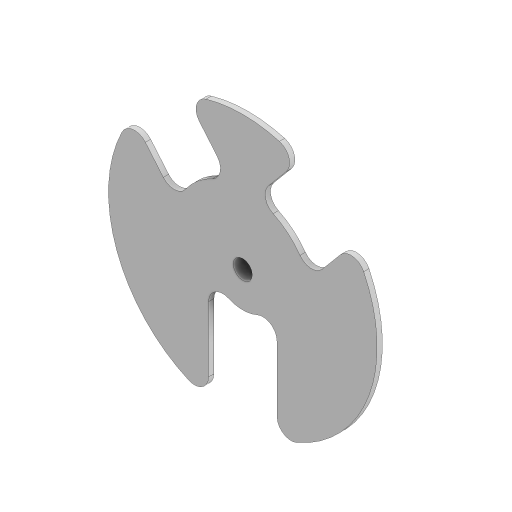
# Autodesk Inventor part: LED Diffuser
Saved by Autodesk Inventor 2024 (Build 280153000, 153)
## iProperties
Created: 2025-04-26
Part Number: LED Diffuser
Material: Generic
Document SubType Name: Modeling
Designer: Binara
Density: 1 g/cm^3
Appearance: Default
Author: Binara
Autodesk Inventor part; units mm, degrees
ref_plane "YZ Plane" through (0, 0, 0) normal (1, 0, 0) x (0, 1, 0)
ref_plane "XZ Plane" through (0, 0, 0) normal (0, 1, 0) x (-1, 0, 0)
ref_plane "XY Plane" through (0, 0, 0) normal (0, 0, 1) x (1, 0, 0)
sketch "Sketch1" plane through (0, 0, 0) normal (0, 0, 1) x (1, 0, 0)
  arc A0 (7.3638, -36.4581) -> (12.7537, -40.2088) centre (11.3638, -36.4581) ccw
  arc A1 (12.7537, -40.2088) -> (35.5951, 21.83) centre (-2.3616, 0.5806) ccw
  arc A2 (35.5951, 21.83) -> (29.0406, 22.4471) centre (32.1048, 19.876) ccw
  line L0 (29.0406, 22.4471) -> (20.2358, 11.954)
  arc A3 (13.9161, 12.201) -> (20.2358, 11.954) centre (17.1717, 14.5251) ccw
  arc A4 (13.9161, 12.201) -> (6.2557, 18.6289) centre (-2.3616, 0.5806) ccw
  arc A5 (4.9149, 24.8097) -> (6.2557, 18.6289) centre (7.9791, 22.2386) ccw
  line L1 (4.9149, 24.8097) -> (13.7198, 35.3029)
  arc A6 (13.7198, 35.3029) -> (11.9738, 41.6506) centre (10.6556, 37.874) ccw
  arc A7 (11.9738, 41.6506) -> (-16.6971, 41.6506) centre (-2.3616, 0.5806) ccw
  arc A8 (-16.6971, 41.6506) -> (-18.443, 35.3029) centre (-15.3789, 37.874) ccw
  line L2 (-18.443, 35.3029) -> (-9.6382, 24.8097)
  arc A9 (-10.979, 18.6289) -> (-9.6382, 24.8097) centre (-12.7024, 22.2386) ccw
  arc A10 (-10.979, 18.6289) -> (-18.6394, 12.201) centre (-2.3616, 0.5806) ccw
  arc A11 (-24.9591, 11.954) -> (-18.6394, 12.201) centre (-21.8949, 14.5251) ccw
  line L3 (-24.9591, 11.954) -> (-33.7639, 22.4471)
  arc A12 (-33.7639, 22.4471) -> (-40.3184, 21.83) centre (-36.8281, 19.876) ccw
  arc A13 (-40.3184, 21.83) -> (-17.477, -40.2088) centre (-2.3616, 0.5806) ccw
  arc A14 (-17.477, -40.2088) -> (-12.0871, -36.4581) centre (-16.0871, -36.4581) ccw
  line L4 (-12.0871, -36.4581) -> (-12.0871, -12.1952)
  arc A15 (-6.4512, -8.5449) -> (-12.0871, -12.1952) centre (-8.0871, -12.1952) ccw
  arc A16 (-6.4512, -8.5449) -> (1.7279, -8.5449) centre (-2.3616, 0.5806) ccw
  arc A17 (7.3638, -12.1952) -> (1.7279, -8.5449) centre (3.3638, -12.1952) ccw
  line L5 (7.3638, -12.1952) -> (7.3638, -36.4581)
  circle A18 centre (-2.3616, 0.5806) radius 2.7
  circle A19 centre (29.9741, 13.9745) radius 2.6
  circle A20 centre (32.6384, 0.5806) radius 2.6
  circle A21 centre (29.9741, -12.8133) radius 2.6
  circle A22 centre (22.3871, -24.1682) radius 2.6
  circle A23 centre (11.0323, -31.7552) radius 2.6
  circle A24 centre (-34.6974, 13.9745) radius 2.6
  circle A25 centre (-37.3616, 0.5806) radius 2.6
  circle A26 centre (-34.6974, -12.8133) radius 2.6
  circle A27 centre (-27.1104, -24.1682) radius 2.6
  circle A28 centre (-15.7556, -31.7552) radius 2.6
  circle A29 centre (-2.3616, 35.5806) radius 2.6
  circle A30 centre (-2.3616, 0.5806) radius 38.1814
  point P0 (0, 0)
  point P1 (7.3638, -36.3414)
  point P2 (28.9846, 22.3804)
  point P3 (13.6637, 35.2361)
  point P4 (-18.387, 35.2361)
  point P5 (-33.7079, 22.3804)
  point P6 (-12.0871, -36.3414)
  constraints: 36 point on circle, 31 centre point, 12 end point, 1 coincident
extrude "Extrusion1" add sketch "Sketch1" along normal blind 1.5 contours L5 A17 A16 A15 L4 A30 L3 A11 A10 A9 L2 L1 A5 A4 A3 L0 | A19 | A20 | A21 | A22 | A23 | A24 | A25 | A26 | A27 | A28 | A29
fillet "Fillet1" radius 4 6 edges at (13.6637, 35.2361, 0.75) (28.9846, 22.3804, 0.75) (7.3638, -36.3414, 0.75) (-12.0871, -36.3414, 0.75) (-18.387, 35.2361, 0.75) (-33.7079, 22.3804, 0.75)
sketch "Sketch2" plane through (0, 0, 0) normal (0, 0, -1) x (-1, 0, 0)
  circle A0 centre (2.3616, 0.5806) radius 2.7 projected
  circle A1 centre (2.3616, 0.5806) radius 7.0777
  point P0 (0, 0)
  constraints: 1 centre point, 1 coincident
extrude "Extrusion2" add sketch "Sketch2" along normal blind 6
body "Solid1"
